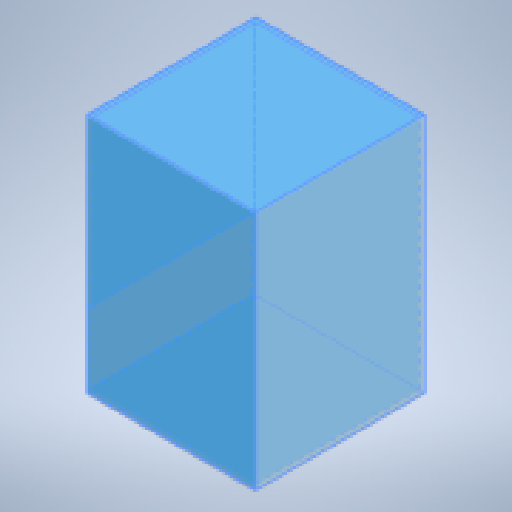
# Autodesk Inventor part: Hot Box Case
Saved by Autodesk Inventor 2023 (Build 270158000, 158)
## iProperties
Created: 2022-08-07
Part Number: Hot Box Case
Material: Polycarbonate, Smoke
Document SubType Name: Modeling
Designer: techv
Density: 1.2 g/cm^3
Appearance: Polycarbonate - Smoked
Author: techv
Autodesk Inventor part; units mm, degrees
ref_plane "YZ Plane" through (0, 0, 0) normal (1, 0, 0) x (0, 1, 0)
ref_plane "XZ Plane" through (0, 0, 0) normal (0, 1, 0) x (-1, 0, 0)
ref_plane "XY Plane" through (0, 0, 0) normal (0, 0, 1) x (1, 0, 0)
sketch "Sketch1" plane through (0, 0, 0) normal (0, 1, 0) x (-1, 0, 0)
  line L0 (-106, 106) -> (106, 106)
  line L1 (106, 106) -> (106, -106)
  line L2 (106, -106) -> (-106, -106)
  line L3 (-106, -106) -> (-106, 106)
  line L4 (-106, 106) -> (106, -106) construction
  line L5 (106, 106) -> (-106, -106) construction
  point P0 (0, 0)
  dimension "d0" = 212
  dimension "d1" = 212
  constraints: 12 end point, 2 midpoint, 2 parallel, 1 horizontal, 1 perpendicular
  measures "d0" distance of L1.end L2.end
  measures "d1" distance of L0.end L1.end
extrude "Extrusion1" add sketch "Sketch1" along normal blind 3
sketch "Sketch2" plane through (0, 3, 0) normal (0, 1, 0) x (1, 0, 0)
  line L0 (-106, 106) -> (-106, -106) projected
  line L1 (106, 106) -> (-106, 106) projected
  line L2 (-106, -106) -> (-103, -106)
  line L3 (-103, -106) -> (-103, 106)
  line L4 (-103, 106) -> (-106, 106)
  line L5 (-106, 106) -> (-106, -106)
  line L6 (106, -106) -> (106, 106) projected
  line L7 (-106, -106) -> (106, -106) projected
  line L8 (106, 106) -> (103, 106)
  line L9 (103, 106) -> (103, -106)
  line L10 (103, -106) -> (106, -106)
  line L11 (106, -106) -> (106, 106)
  line L12 (106, 106) -> (-106, 106)
  line L13 (-106, 106) -> (-106, 103)
  line L14 (-106, 103) -> (106, 103)
  line L15 (106, 103) -> (106, 106)
  line L16 (-106, -106) -> (106, -106)
  line L17 (106, -106) -> (106, -103)
  line L18 (106, -103) -> (-106, -103)
  line L19 (-106, -103) -> (-106, -106)
  point P0 (0, 0)
  point P1 (-103, 103)
  point P2 (103, 103)
  point P3 (103, -103)
  point P4 (-103, -103)
  dimension "d4" = 3
  dimension "d5" = 3
  dimension "d6" = 3
  dimension "d7" = 3
  constraints: 32 end point, 8 parallel, 4 horizontal, 4 perpendicular, 4 point on line
  measures "d4" distance of L4.end L3.end
  measures "d5" distance of L10.end L9.end
  measures "d6" distance of L13.end L12.end
  measures "d7" distance of L17.end L16.end
extrude "Extrusion2" add sketch "Sketch2" along normal blind 300 contours L1 L3 L14 L0 | L14 L3 L18 L0 | L1 L9 L14 L3 | L18 L3 L2 L0 | L1 L6 L14 L9 | L18 L9 L7 L3 | L14 L6 L18 L9 | L18 L6 L7 L9
sketch "Sketch3" plane through (-103, 3, 103) normal (1, 0, 0) x (0, 0, -1)
  line L0 (0, 0) -> (0, 300) projected
  line L1 (206, 0) -> (206, 300) projected
  line L2 (0, 300) -> (206, 300)
  line L3 (206, 300) -> (206, 297)
  line L4 (206, 297) -> (0, 297)
  line L5 (0, 297) -> (0, 300)
  point P0 (103, -3)
  dimension "d10" = 3
  constraints: 8 end point, 2 parallel, 1 horizontal, 1 perpendicular, 1 point on line
  measures "d10" distance of L2.end L3.end
extrude "Extrusion3" add sketch "Sketch3" along normal up to surface (209 mm away)
sketch "Sketch4" plane through (-106, 0, -106) normal (-1, 0, 0) x (0, 0, 1)
  line L0 (3, 3) -> (209, 3) projected
  line L1 (3, 3) -> (209, 3)
  line L2 (209, 3) -> (209, 93)
  line L3 (209, 93) -> (3, 93)
  line L4 (3, 93) -> (3, 3)
  point P0 (106, 0)
  dimension "d13" = 90
  constraints: 8 end point, 2 parallel, 1 horizontal, 1 perpendicular
  measures "d13" distance of L2.end L1.end
extrude "Extrusion4" cut sketch "Sketch4" against normal blind 10
sketch "Sketch5" plane through (-106, 0, 106) normal (0, 0, 1) x (1, 0, 0)
  line L0 (0, 93) -> (3, 93) projected
  line L1 (0, 3) -> (209, 3) projected
  line L2 (0, 93) -> (209, 93)
  line L3 (209, 93) -> (209, 3)
  line L4 (209, 3) -> (0, 3)
  line L5 (0, 3) -> (0, 93)
  point P0 (106, 0)
  constraints: 8 end point, 2 parallel, 1 horizontal, 1 perpendicular
extrude "Extrusion5" cut sketch "Sketch5" against normal blind 10
sketch "Sketch6" plane through (106, 0, 106) normal (1, 0, 0) x (0, 0, -1)
  line L0 (3, 93) -> (209, 93) projected
  line L1 (0, 303) -> (212, 303) projected
  line L2 (0, 0) -> (0, 303) projected
  line L3 (0, 0) -> (212, 0) projected
  line L4 (212, 0) -> (212, 303) projected
  line L5 (212, 0) -> (0, 0)
  line L6 (0, 0) -> (0, 93)
  line L7 (0, 93) -> (212, 93)
  line L8 (212, 93) -> (212, 0)
  line L9 (212, 93) -> (0, 0) construction
  line L10 (0, 93) -> (0, 3) construction
  line L11 (0, 93) -> (212, 0) construction
  line L12 (131, 71.5) -> (81, 71.5)
  line L13 (81, 71.5) -> (81, 21.5)
  line L14 (81, 21.5) -> (131, 21.5)
  line L15 (131, 21.5) -> (131, 71.5)
  line L16 (131, 71.5) -> (81, 21.5) construction
  line L17 (81, 71.5) -> (131, 21.5) construction
  point P0 (106, 0)
  point P1 (106, 46.5)
  dimension "d18" = 50
  dimension "d19" = 50
  constraints: 24 end point, 4 parallel, 3 midpoint, 2 horizontal, 2 perpendicular, 1 point on line
  measures "d18" distance of L14.end L13.end
  measures "d19" distance of L13.end L12.end
extrude "Extrusion6" cut sketch "Sketch6" against normal blind 10 contours L15 L14 L13 L12
body "Solid1"
